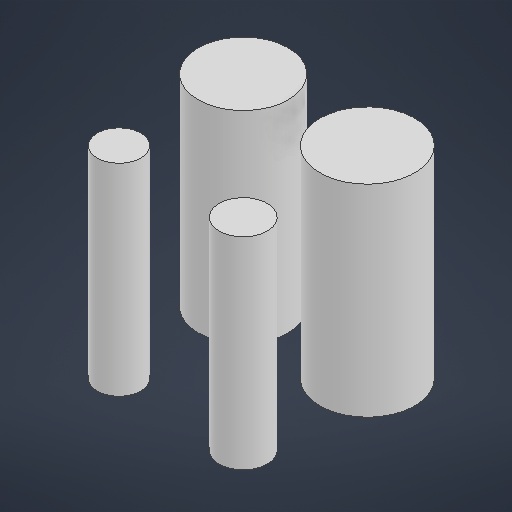
# Autodesk Inventor part: klinyrozne
Saved by Autodesk Inventor 2026.2 (Build 302298010, 298A)
## iProperties
Created: 2026-05-14
Part Number: klinyrozne
Material: Ogólny
Document SubType Name: Modeling
Designer: karol
Density: 1 g/cm^3
Appearance: Domyślna
Author: karol
Autodesk Inventor part; units mm, degrees
ref_plane "YZ Plane" through (0, 0, 0) normal (1, 0, 0) x (0, 1, 0)
ref_plane "XZ Plane" through (0, 0, 0) normal (0, 1, 0) x (-1, 0, 0)
ref_plane "XY Plane" through (0, 0, 0) normal (0, 0, 1) x (1, 0, 0)
sketch "Szkic1" plane through (0, 0, 0) normal (0, 1, 0) x (-1, 0, 0)
  circle A0 centre (0, 0) radius 0.7
  circle A1 centre (0, -4) radius 1.45
  circle A2 centre (-4, 0) radius 0.775
  circle A3 centre (-4, -4) radius 1.525
  line L0 (0, 0) -> (-4, 0)
  line L1 (-4, 0) -> (-4, -4)
  dimension "d0" = 1.4
  dimension "d1" = 2.9
  dimension "d2" = 4
  dimension "d5" = 1.55
  dimension "d6" = 3.05
  dimension "d7" = 4
  dimension "d8" = 4
  dimension "d9" = 4
  constraints: 4 centre point, 4 end point, 1 coincident, 1 horizontal, 1 perpendicular
  measures "d0" diameter of A0
  measures "d1" diameter of A1
  measures "d2" distance of point (0, 0) A1.centre
  measures "d5" diameter of A2
  measures "d6" diameter of A3
  measures "d7" distance of L0.end L1.end
  measures "d8" distance of L0.end point (0, 0)
  measures "d9" distance of A1.centre L1.end
extrude "Wyciągnięcie proste1" add sketch "Szkic1" along normal blind 6.5
